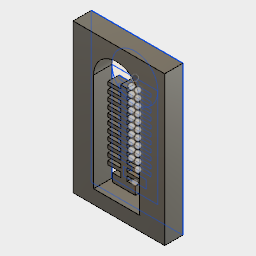
One-finger_mold v8 (Autodesk Fusion 360 design; units mm, degrees)
Autodesk Fusion 360 part; units mm, degrees
sketch "Sketch1" plane through (0, 0, 0) normal (0, 0, 1) x (1, 0, 0)
  line L0 (-11, -3.9565) -> (9, -3.9565)
  line L1 (9, -3.9565) -> (9, 39.0435)
  line L2 (9, 39.0435) -> (-11, 39.0435)
  line L3 (-11, 39.0435) -> (-11, -3.9565)
  circle A0 centre (-1, 39.0435) radius 10
  line L4 (-1, -3.9565) -> (-1, 39.0435) construction
  line L5 (-8, 5.0435) -> (-8, 6.5435)
  line L6 (-8, 6.5435) -> (-2.4, 6.5435)
  line L7 (-2.4, 6.5435) -> (-2.4, 8.0435)
  line L8 (-8, 5.0435) -> (-2.4, 5.0435)
  line L9 (-8, 8.0435) -> (-2.4, 8.0435)
  line L10 (-8, 9.5435) -> (-2.4, 9.5435)
  line L11 (-8, 8.0435) -> (-8, 9.5435)
  line L12 (-2.4, 9.5435) -> (-2.4, 11.0435)
  line L13 (-8, 11.0435) -> (-2.4, 11.0435)
  line L14 (-8, 12.5435) -> (-2.4, 12.5435)
  line L15 (-8, 11.0435) -> (-8, 12.5435)
  line L16 (-2.4, 12.5435) -> (-2.4, 14.0435)
  line L17 (-8, 14.0435) -> (-2.4, 14.0435)
  line L18 (-8, 15.5435) -> (-2.4, 15.5435)
  line L19 (-8, 14.0435) -> (-8, 15.5435)
  line L20 (-2.4, 15.5435) -> (-2.4, 17.0435)
  line L21 (-8, 17.0435) -> (-2.4, 17.0435)
  line L22 (-8, 18.5435) -> (-2.4, 18.5435)
  line L23 (-8, 17.0435) -> (-8, 18.5435)
  line L24 (-2.4, 18.5435) -> (-2.4, 20.0435)
  line L25 (-8, 20.0435) -> (-2.4, 20.0435)
  line L26 (-8, 21.5435) -> (-2.4, 21.5435)
  line L27 (-8, 20.0435) -> (-8, 21.5435)
  line L28 (-2.4, 21.5435) -> (-2.4, 23.0435)
  line L29 (-8, 23.0435) -> (-2.4, 23.0435)
  line L30 (-8, 24.5435) -> (-2.4, 24.5435)
  line L31 (-8, 23.0435) -> (-8, 24.5435)
  line L32 (-2.4, 24.5435) -> (-2.4, 26.0435)
  line L33 (-8, 26.0435) -> (-2.4, 26.0435)
  line L34 (-8, 27.5435) -> (-2.4, 27.5435)
  line L35 (-8, 26.0435) -> (-8, 27.5435)
  line L36 (-2.4, 27.5435) -> (-2.4, 29.0435)
  line L37 (-8, 29.0435) -> (-2.4, 29.0435)
  line L38 (-8, 30.5435) -> (-2.4, 30.5435)
  line L39 (-8, 29.0435) -> (-8, 30.5435)
  line L40 (-2.4, 30.5435) -> (-2.4, 32.0435)
  line L41 (-8, 32.0435) -> (-2.4, 32.0435)
  line L42 (-8, 33.5435) -> (-2.4, 33.5435)
  line L43 (-8, 32.0435) -> (-8, 33.5435)
  line L44 (-2.4, 33.5435) -> (-2.4, 35.0435)
  line L45 (-8, 35.0435) -> (-2.4, 35.0435)
  line L46 (-8, 36.5435) -> (-2.4, 36.5435)
  line L47 (-8, 35.0435) -> (-8, 36.5435)
  line L48 (-2.4, 36.5435) -> (-2.4, 38.0435)
  line L49 (0.4, 36.5435) -> (0.4, 38.0435)
  line L50 (6, 29.0435) -> (6, 30.5435)
  line L51 (6, 30.5435) -> (0.4, 30.5435)
  line L52 (6, 29.0435) -> (0.4, 29.0435)
  line L53 (0.4, 27.5435) -> (0.4, 29.0435)
  line L54 (6, 26.0435) -> (6, 27.5435)
  line L55 (6, 27.5435) -> (0.4, 27.5435)
  line L56 (6, 26.0435) -> (0.4, 26.0435)
  line L57 (0.4, 24.5435) -> (0.4, 26.0435)
  line L58 (6, 23.0435) -> (6, 24.5435)
  line L59 (6, 24.5435) -> (0.4, 24.5435)
  line L60 (6, 23.0435) -> (0.4, 23.0435)
  line L61 (0.4, 21.5435) -> (0.4, 23.0435)
  line L62 (6, 20.0435) -> (6, 21.5435)
  line L63 (6, 21.5435) -> (0.4, 21.5435)
  line L64 (6, 20.0435) -> (0.4, 20.0435)
  line L65 (0.4, 18.5435) -> (0.4, 20.0435)
  line L66 (6, 17.0435) -> (6, 18.5435)
  line L67 (6, 18.5435) -> (0.4, 18.5435)
  line L68 (6, 17.0435) -> (0.4, 17.0435)
  line L69 (0.4, 15.5435) -> (0.4, 17.0435)
  line L70 (6, 15.5435) -> (0.4, 15.5435)
  line L71 (6, 14.0435) -> (6, 15.5435)
  line L72 (6, 14.0435) -> (0.4, 14.0435)
  line L73 (0.4, 12.5435) -> (0.4, 14.0435)
  line L74 (6, 11.0435) -> (6, 12.5435)
  line L75 (6, 12.5435) -> (0.4, 12.5435)
  line L76 (6, 11.0435) -> (0.4, 11.0435)
  line L77 (0.4, 9.5435) -> (0.4, 11.0435)
  line L78 (6, 8.0435) -> (6, 9.5435)
  line L79 (6, 9.5435) -> (0.4, 9.5435)
  line L80 (6, 8.0435) -> (0.4, 8.0435)
  line L81 (6, 5.0435) -> (0.4, 5.0435)
  line L82 (0.4, 6.5435) -> (0.4, 8.0435)
  line L83 (6, 6.5435) -> (0.4, 6.5435)
  line L84 (6, 5.0435) -> (6, 6.5435)
  line L85 (6, 33.5435) -> (0.4, 33.5435)
  line L86 (6, 32.0435) -> (6, 33.5435)
  line L87 (0.4, 33.5435) -> (0.4, 35.0435)
  line L88 (6, 35.0435) -> (0.4, 35.0435)
  line L89 (6, 36.5435) -> (0.4, 36.5435)
  line L90 (6, 35.0435) -> (6, 36.5435)
  line L91 (6, 32.0435) -> (0.4, 32.0435)
  line L92 (0.4, 30.5435) -> (0.4, 32.0435)
  line L93 (-2.4, 38.0435) -> (0.4, 38.0435)
  line L94 (-2.4, 5.0435) -> (-2.4, 3)
  line L95 (-2.4, 3) -> (-6, 3)
  line L96 (-6, 3) -> (-6, -0.5877)
  line L97 (-6, -0.5877) -> (-1, -0.5877)
  line L98 (0.4, 3) -> (4, 3)
  line L99 (0.4, 5.0435) -> (0.4, 3)
  line L100 (4, 3) -> (4, -0.5877)
  line L101 (4, -0.5877) -> (-1, -0.5877)
  line L102 (-20, -10) -> (20, -10)
  line L103 (20, -10) -> (20, 55)
  line L104 (20, 55) -> (-20, 55)
  line L105 (-20, 55) -> (-20, -10)
  dimension "d1" = 20
  dimension "d6" = 43
  dimension "d8" = 1.5
  dimension "d9" = 5.6
  dimension "d10" = 1.5
  dimension "d14" = 8.5
  dimension "d15" = 3
  dimension "d16" = 9
  measures "d1" distance of L0.start L0.end
  measures "d6" distance of L0.end L1.end
  measures "d8" distance of L5.start L5.end
  measures "d9" distance of L5.end L6.end
  measures "d10" distance of L6.end L7.end
  measures "d16" distance of L0 L8
extrude "Extrude1" add sketch "Sketch1" along normal blind 8 makes body 1
extrude "Extrude2" add sketch "Sketch1" along normal blind 4.8 separate body contours A0 L38 L40 L41 L42 L43 L44 L45 L46 L47 L48 L49 L51 L85 L86 L87 L88 L89 L90 L91 L92 L93 | A0 L5 L6 L7 L8 L9 L10 L11 L12 L13 L14 L15 L16 L17 L18 L19 L20 L21 L22 L23 L24 L25 L26 L27 L28 L29 L30 L31 L32 L33 L34 L35 L36 L37 L38 L39 L50 L51 L52 L53 L54 L55 L56 L57 L58 L59 L60 L61 L62 L63 L64 L65 L66 L67 L68 L69 L70 L71 L72 L73 L74 L75 L76 L77 L78 L79 L80 L81 L82 L83 L84 L94 L95 L96 L97 L98 L99 L100 L101 makes body 2
equation "d1 = mold_width"
equation "mold_width = 20 mm"
equation "mold_length = 43 mm"
equation "comb_width = 7 mm"
equation "comb_tooth_width = 1.5 mm"
equation "d6 = mold_length"
equation "d8 = comb_tooth_width"
equation "d9 = comb_width * 0.8"
equation "d10 = comb_tooth_width"
equation "d16 = 6 * comb_tooth_width"
equation "mold_depth = 8 mm"
equation "d18 = mold_depth"
equation "d20 = 0.6 * mold_depth"
